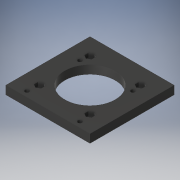
# Autodesk Inventor part: lidarMount
Saved by Autodesk Inventor 2017 (Build 210142000, 142)
## iProperties
Created: 2017-03-03
Part Number: lidarMount
Material: Generic
Document SubType Name: Modeling
Designer: Naga
Density: 1 g/cm^3
Appearance: Smooth - Black
Author: Naga
Autodesk Inventor part; units mm, degrees
ref_plane "YZ Plane" through (0, 0, 0) normal (1, 0, 0) x (0, 1, 0)
ref_plane "XZ Plane" through (0, 0, 0) normal (0, 1, 0) x (-1, 0, 0)
ref_plane "XY Plane" through (0, 0, 0) normal (0, 0, 1) x (1, 0, 0)
sketch "Sketch1" plane through (0, 0, 0) normal (0, 1, 0) x (-1, 0, 0)
  line L0 (0, 0) -> (63.5, 0)
  line L1 (63.5, 0) -> (63.5, -63.5)
  line L2 (63.5, -63.5) -> (0, -63.5)
  line L3 (0, -63.5) -> (0, 0)
  line L4 (0, -31.75) -> (31.75, -31.75)
  line L5 (31.75, -31.75) -> (31.75, -63.5)
  line L6 (31.75, -31.75) -> (12.7, -31.75)
  line L7 (31.75, -31.75) -> (50.8, -31.75) construction
  line L8 (12.7, -31.75) -> (12.7, -50.8)
  circle A0 centre (12.7, -50.8) radius 1.5875
  circle A1 centre (50.8, -50.8) radius 1.5875
  circle A2 centre (12.7, -12.7) radius 1.5875
  circle A3 centre (50.8, -12.7) radius 1.5875
  dimension "d0" = 63.5
  dimension "d1" = 63.5
  dimension "d2" = 19.05
  dimension "d3" = 180
  dimension "d4" = 19.05
  dimension "d5" = 3.175
  dimension "d8" = 38.1
  dimension "d11" = 38.1
  constraints: 18 end point, 4 centre point, 4 horizontal, 3 parallel, 2 midpoint, 2 vertical, 1 coincident, 1 collinear, 1 perpendicular, 6 other
  measures "d0" distance of L1.end L2.end
  measures "d1" distance of L0.end L1.end
  measures "d2" distance of L4.end L6.end
  measures "d3" angle of L6 L7
  measures "d4" distance of L6.end L8.end
  measures "d5" diameter of A0
  measures "d8" distance of A0.centre A1.centre
  measures "d11" distance of A0.centre A2.centre
extrude "Extrusion1" add sketch "Sketch1" along normal blind 3.175
sketch "Sketch2" plane through (0, 3.175, 0) normal (0, 1, 0) x (1, 0, 0)
  circle A0 centre (-12.7, 12.7) radius 1.5875 projected
  line L0 (-12.7, 15.875) -> (-9.9504, 14.2875)
  line L1 (-9.9504, 14.2875) -> (-9.9504, 11.1125)
  line L2 (-9.9504, 11.1125) -> (-12.7, 9.525)
  line L3 (-12.7, 9.525) -> (-15.4496, 11.1125)
  line L4 (-15.4496, 11.1125) -> (-15.4496, 14.2875)
  line L5 (-15.4496, 14.2875) -> (-12.7, 15.875)
  circle A1 centre (-50.8, 12.7) radius 1.5875 projected
  circle A2 centre (-12.7, 12.7) radius 1.5875 projected
  circle A3 centre (-50.8, 50.8) radius 1.5875 projected
  circle A4 centre (-12.7, 50.8) radius 1.5875 projected
  line L6 (0, 63.5) -> (-63.5, 63.5) projected
  line L7 (-63.5, 63.5) -> (-63.5, 0) projected
  line L8 (-63.5, 0) -> (0, 0) projected
  line L9 (0, 0) -> (0, 63.5) projected
  line L10 (-50.8, 15.875) -> (-48.0504, 14.2875)
  line L11 (-48.0504, 11.1125) -> (-50.8, 9.525)
  line L12 (-50.8, 9.525) -> (-53.5496, 11.1125)
  line L13 (-53.5496, 11.1125) -> (-53.5496, 14.2875)
  line L14 (-53.5496, 14.2875) -> (-50.8, 15.875)
  line L15 (-48.0504, 14.2875) -> (-48.0504, 11.1125)
  line L16 (-12.7, 53.975) -> (-9.9504, 52.3875)
  line L17 (-9.9504, 49.2125) -> (-12.7, 47.625)
  line L18 (-12.7, 47.625) -> (-15.4496, 49.2125)
  line L19 (-15.4496, 49.2125) -> (-15.4496, 52.3875)
  line L20 (-15.4496, 52.3875) -> (-12.7, 53.975)
  line L21 (-9.9504, 52.3875) -> (-9.9504, 49.2125)
  line L22 (-50.8, 53.975) -> (-48.0504, 52.3875)
  line L23 (-48.0504, 49.2125) -> (-50.8, 47.625)
  line L24 (-50.8, 47.625) -> (-53.5496, 49.2125)
  line L25 (-53.5496, 49.2125) -> (-53.5496, 52.3875)
  line L26 (-53.5496, 52.3875) -> (-50.8, 53.975)
  line L27 (-48.0504, 52.3875) -> (-48.0504, 49.2125)
  dimension "d16" = 6.35
  dimension "d19" = 38.1
  dimension "d22" = 38.1
  constraints: 48 end point, 1 coincident, 1 horizontal, 1 vertical, 52 other
  measures "d16" distance of L2.end L0.start
  measures "d19" distance of point (-12.7, 12.7) point (-50.8, 12.7)
  measures "d22" distance of point (-12.7, 12.7) point (-12.7, 50.8)
extrude "Extrusion2" add sketch "Sketch2" along normal blind 3.175 contours L9 L8 L7 L6
sketch "Sketch4" plane through (0, 6.35, 0) normal (0, 1, 0) x (1, 0, 0)
  line L0 (-31.75, 24.13) -> (-31.75, 0)
  line L1 (-31.75, 24.13) -> (-11.7475, 24.13)
  line L2 (-11.7475, 24.13) -> (-11.7475, 44.1325)
  circle A0 centre (-11.7475, 44.1325) radius 1.5875
  circle A1 centre (-51.7525, 44.1325) radius 1.5875
  circle A2 centre (-11.7475, 4.1275) radius 1.5875
  circle A3 centre (-51.7525, 4.1275) radius 1.5875
  circle A4 centre (-11.7475, 44.1325) radius 2.3812
  point P0 (0, 0)
  dimension "d41" = 20.0025
  dimension "d42" = 24.13
  dimension "d43" = 3.175
  dimension "d44" = 40.005
  dimension "d45" = 40.005
  dimension "d46" = 4.7625
  constraints: 6 end point, 5 centre point, 2 coincident, 2 vertical, 1 horizontal, 6 other
  measures "d41" distance of L0.start L1.end
  measures "d42" distance of L0.start L0.end
  measures "d43" diameter of A0
  measures "d44" distance of A0.centre A1.centre
  measures "d45" distance of A0.centre A2.centre
  measures "d46" diameter of A4
extrude "Extrusion3" cut sketch "Sketch4" against normal up to surface (6.35 mm away) contours A0 | A1 | A2 | A3
sketch "Sketch5" plane through (0, 0, 0) normal (0, -1, 0) x (1, 0, 0)
  circle A0 centre (-51.7525, -4.1275) radius 1.5875 projected
  circle A1 centre (-11.7475, -4.1275) radius 1.5875 projected
  circle A2 centre (-51.7525, -44.1325) radius 1.5875 projected
  circle A3 centre (-11.7475, -44.1325) radius 1.5875 projected
  circle A4 centre (-51.7525, -4.1275) radius 2.3813
  circle A5 centre (-51.7525, -44.1325) radius 2.3812
  circle A6 centre (-11.7475, -44.1325) radius 2.3812
  circle A7 centre (-11.7475, -4.1275) radius 2.3812
  point P0 (0, 0)
  dimension "d51" = 4.7625
  dimension "d52" = 4.7625
  dimension "d53" = 4.7625
  dimension "d54" = 4.7625
  constraints: 4 centre point, 4 coincident
  measures "d51" diameter of A4
  measures "d52" diameter of A5
  measures "d53" diameter of A6
  measures "d54" diameter of A7
extrude "Extrusion4" cut sketch "Sketch5" against normal blind 3.175 contours A0 | A1 | A2 | A3 | A4 | A5 | A6 | A7
sketch "Sketch6" plane through (0, 6.35, 0) normal (0, 1, 0) x (1, 0, 0)
  circle A0 centre (-51.7525, 4.1275) radius 1.5875 projected
  circle A1 centre (-11.7475, 44.1325) radius 1.5875 projected
  circle A2 centre (-11.7475, 4.1275) radius 1.5875 projected
  circle A3 centre (-51.7525, 44.1325) radius 1.5875 projected
  line L0 (-48.0504, 52.3875) -> (-48.0504, 49.2125) projected
  line L1 (-48.0504, 49.2125) -> (-50.8, 47.625) projected
  line L2 (-50.8, 47.625) -> (-53.5496, 49.2125) projected
  line L3 (-53.5496, 49.2125) -> (-53.5496, 52.3875) projected
  line L4 (-53.5496, 52.3875) -> (-50.8, 53.975) projected
  line L5 (-50.8, 53.975) -> (-48.0504, 52.3875) projected
  line L6 (-9.9504, 52.3875) -> (-9.9504, 49.2125) projected
  line L7 (-9.9504, 49.2125) -> (-12.7, 47.625) projected
  line L8 (-12.7, 47.625) -> (-15.4496, 49.2125) projected
  line L9 (-15.4496, 49.2125) -> (-15.4496, 52.3875) projected
  line L10 (-15.4496, 52.3875) -> (-12.7, 53.975) projected
  line L11 (-12.7, 53.975) -> (-9.9504, 52.3875) projected
  line L12 (-48.0504, 14.2875) -> (-48.0504, 11.1125) projected
  line L13 (-48.0504, 11.1125) -> (-50.8, 9.525) projected
  line L14 (-50.8, 9.525) -> (-53.5496, 11.1125) projected
  line L15 (-53.5496, 11.1125) -> (-53.5496, 14.2875) projected
  line L16 (-53.5496, 14.2875) -> (-50.8, 15.875) projected
  line L17 (-50.8, 15.875) -> (-48.0504, 14.2875) projected
  line L18 (-9.9504, 14.2875) -> (-9.9504, 11.1125) projected
  line L19 (-9.9504, 11.1125) -> (-12.7, 9.525) projected
  line L20 (-12.7, 9.525) -> (-15.4496, 11.1125) projected
  line L21 (-15.4496, 11.1125) -> (-15.4496, 14.2875) projected
  line L22 (-15.4496, 14.2875) -> (-12.7, 15.875) projected
  line L23 (-12.7, 15.875) -> (-9.9504, 14.2875) projected
  line L24 (0, 63.5) -> (-63.5, 63.5) projected
  line L25 (-63.5, 63.5) -> (-63.5, 0) projected
  line L26 (-63.5, 0) -> (0, 0) projected
  line L27 (0, 0) -> (0, 63.5) projected
  circle A4 centre (-31.75, 31.75) radius 19.0514
  constraints: 1 centre point
extrude "Extrusion5" cut sketch "Sketch6" against normal up to surface (6.35 mm away) contours A4
body "Solid1"
